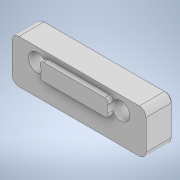
# Autodesk Inventor part: SideHolderFix2
Saved by Autodesk Inventor 2021 (Build 250183000, 183)
## iProperties
Created: 2020-11-09
Part Number: SideHolderFix2
Material: Generic
Document SubType Name: Modeling
Designer: Viktor
Density: 1 g/cm^3
Appearance: Default
Author: Viktor
## iProperties of the stored document _3DPrint.ipt
Created: 2020-11-09
Part Number: _3DPrint
Material: Generic
Document SubType Name: Modeling
Designer: Viktor
Density: 1 g/cm^3
Appearance: Default
Author: Viktor
Autodesk Inventor part; units mm, degrees
ref_plane "YZ Plane" through (0, 0, 0) normal (1, 0, 0) x (0, 1, 0)
ref_plane "XZ Plane" through (0, 0, 0) normal (0, 1, 0) x (-1, 0, 0)
ref_plane "XY Plane" through (0, 0, 0) normal (0, 0, 1) x (1, 0, 0)
sketch "Sketch1" plane through (0, 0, 0) normal (0, 0, 1) x (1, 0, 0)
  line L0 (-20, -4) -> (20, -4)
  line L1 (20, -4) -> (20, 4)
  line L2 (20, 4) -> (-20, 4)
  line L3 (-20, 4) -> (-20, -4)
  line L4 (-20, -4) -> (20, 4) construction
  line L5 (20, -4) -> (-20, 4) construction
  point P0 (0, 0)
  dimension "d0" = 8
  dimension "d1" = 40
  constraints: 12 end point, 2 midpoint, 2 parallel, 1 horizontal, 1 perpendicular
  measures "d0" distance between parallel lines of L0 L2
  measures "d1" distance between parallel lines of L1 L3
extrude "Extrusion1" add sketch "Sketch1" along normal blind 8
sketch "Sketch2" plane through (-20, -4, 0) normal (0, -1, 0) x (1, 0, 0)
  line L0 (0, 0) -> (40, 0) projected
  line L1 (40, 0) -> (40, 8) projected
  line L2 (0, 8) -> (40, 8) projected
  line L3 (0, 0) -> (0, 8) projected
  point P0 (20, 0)
extrude "Extrusion2" add sketch "Sketch2" along normal blind 5
sketch "Sketch3" plane through (0, 0, 8) normal (0, 0, 1) x (1, 0, 0)
  line L0 (-15, -3) -> (15, -3) construction
  line L1 (15, -3) -> (15, 3) construction
  line L2 (15, 3) -> (-15, 3) construction
  line L3 (-15, 3) -> (-15, -3) construction
  line L4 (-15, -3) -> (15, 3) construction
  line L5 (15, -3) -> (-15, 3) construction
  line L6 (-28, 0) -> (28, 0) construction
  circle A0 centre (-12.5, 0) radius 2.65
  line L7 (0, 6.6) -> (0, -11.6) construction
  line L8 (15, 3) -> (15, -3) construction
  circle A1 centre (12.5, 0) radius 2.65
  point P0 (0, 0)
  dimension "d6" = 6
  dimension "d7" = 30
  dimension "d8" = 5.3
  dimension "d20" = 25
  constraints: 14 end point, 2 centre point, 2 midpoint, 2 parallel, 1 horizontal, 1 perpendicular, 1 point on line, 1 symmetric about line, 1 other
  measures "d6" distance of L0.end L1.end
  measures "d7" distance of L0.start L0.end
  measures "d8" diameter of A0
  measures "d20" distance of A1.centre A0.centre
extrude "Extrusion3" cut sketch "Sketch3" against normal through all
sketch "Sketch4" plane through (0, 0, 8) normal (0, 0, 1) x (1, 0, 0)
  line L0 (-13, -2.5) -> (13, -2.5)
  line L1 (13, -2.5) -> (13, 2.5)
  line L2 (13, 2.5) -> (-13, 2.5)
  line L3 (-13, 2.5) -> (-13, -2.5)
  line L4 (-13, -2.5) -> (13, 2.5) construction
  line L5 (13, -2.5) -> (-13, 2.5) construction
  circle A0 centre (-12.5, 0) radius 2.65 projected
  circle A1 centre (12.5, 0) radius 2.65 projected
  point P0 (0, 0)
  point P1 (-8.1211, 2.5)
  point P2 (-8.1211, -2.5)
  point P3 (-11.6211, -2.5)
  point P4 (-11.6211, 2.5)
  point P5 (11.6211, -2.5)
  point P6 (11.6211, 2.5)
  dimension "d11" = 26
  dimension "d12" = 5
  constraints: 12 end point, 2 midpoint, 2 parallel, 1 horizontal, 1 perpendicular
  measures "d11" distance of L1.end L2.end
  measures "d12" distance of L0.end L1.end
extrude "Extrusion4" add sketch "Sketch4" along normal blind 1.5 contours A0 L2 A1 L0
fillet "Fillet1" radius 1 4 edges at (-11.6211, -2.5, 8.75) (-11.6211, 2.5, 8.75) (11.6211, -2.5, 8.75) (11.6211, 2.5, 8.75)
fillet "Fillet2" radius 2 4 edges at (-20, -9, 4) (-20, 4, 4) (20, -9, 4) (20, 4, 4)
chamfer "Chamfer1" distance 0.5 angle 45 6 edges at (0, -9, 0) (20, -2.5, 0) (0, 4, 0) (-20, -2.5, 0) (-15.15, 0, 0) (9.85, 0, 0)
body "Solid1"
